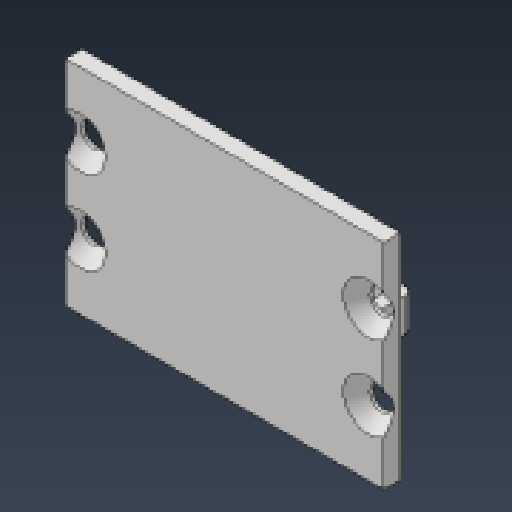
# Autodesk Inventor part: PCBs_Holder
Saved by Autodesk Inventor 2026.2 (Build 302298010, 298A)
## iProperties
Created: 2026-04-14
Part Number: PCBs_Holder
Material: Generic
Document SubType Name: Modeling
Designer: szymo
Density: 1 g/cm^3
Appearance: Default
Author: szymo
Autodesk Inventor part; units mm, degrees
ref_plane "YZ Plane" through (0, 0, 0) normal (1, 0, 0) x (0, 1, 0)
ref_plane "XZ Plane" through (0, 0, 0) normal (0, 1, 0) x (-1, 0, 0)
ref_plane "XY Plane" through (0, 0, 0) normal (0, 0, 1) x (1, 0, 0)
sketch "Sketch1" plane through (0, 0, 0) normal (0, 0, 1) x (1, 0, 0)
  line L0 (19.2, 22.3883) -> (-19.2, 22.3883)
  line L1 (-19, 22.3883) -> (-19, 47.9488)
  line L2 (-19.2, 47.9488) -> (19.2, 47.9488)
  line L3 (19, 47.9488) -> (19, 22.3883)
  line L4 (15, 33.1685) -> (9.5, 33.1685)
  line L5 (9.5, 33.1685) -> (9.5, 37.1685)
  line L6 (9.5, 37.1685) -> (15, 37.1685)
  line L7 (15, 37.1685) -> (15, 33.1685)
  line L8 (-15, 33.1685) -> (-9.5, 33.1685)
  line L9 (-9.5, 33.1685) -> (-9.5, 37.1685)
  line L10 (-9.5, 37.1685) -> (-15, 37.1685)
  line L11 (-15, 37.1685) -> (-15, 33.1685)
  circle A0 centre (-17.2, 40.1685) radius 1.75 projected
  circle A1 centre (-17.2, 30.1685) radius 1.75 projected
  line L12 (-19.2, 22.3883) -> (-15.2, 22.3883) projected
  line L13 (-15.2, 22.3883) -> (-15.2, 47.9488) projected
  line L14 (-19.2, 47.9488) -> (-15.2, 47.9488) projected
  line L15 (-19.2, 22.3883) -> (-19.2, 47.9488) projected
  circle A2 centre (17.2, 40.1685) radius 1.75 projected
  circle A3 centre (17.2, 30.1685) radius 1.75 projected
  line L16 (19.2, 22.3883) -> (15.2, 22.3883) projected
  line L17 (19.2, 22.3883) -> (19.2, 47.9488) projected
  line L18 (19.2, 47.9488) -> (15.2, 47.9488) projected
  line L19 (15.2, 22.3883) -> (15.2, 47.9488) projected
  point P0 (0, 0)
  dimension "d4" = 10.7802
  dimension "d5" = 10.7802
  dimension "d6" = 10.7802
  dimension "d7" = 10.7802
  dimension "d10" = 4
  dimension "d11" = 4
  dimension "d12" = 5.5
  dimension "d13" = 5.5
  dimension "d33" = 0.2
  dimension "d34" = 0.2
  dimension "d43" = 0.2
  dimension "d44" = 0.2
  constraints: 24 end point, 6 parallel, 4 coincident, 3 horizontal, 3 perpendicular, 3 point on line
  measures "d4" distance between parallel lines of L0 L4
  measures "d5" distance between parallel lines of L0 L8
  measures "d6" distance between parallel lines of L2 L6
  measures "d7" distance between parallel lines of L2 L10
  measures "d10" distance between parallel lines of L6 L4
  measures "d11" distance between parallel lines of L10 L8
  measures "d12" distance between parallel lines of L7 L5
  measures "d13" distance between parallel lines of L9 L11
  measures "d33" distance between parallel lines of L13 L11
  measures "d34" distance between parallel lines of L19 L7
  measures "d43" distance between parallel lines of L1 L15
  measures "d44" distance between parallel lines of L17 L3
extrude "Extrusion3" add sketch "Sketch1" against normal blind 2 contours L0 L19 L2 L3 | L0 L13 L2 L19 | L0 L1 L2 L13 | L4 L5 L6 L7 | L11 L10 L9 L8 | A0 | A1 | A2 | A3
extrude "Extrusion4" add sketch "Sketch1" against normal blind 7.5 contours L4 L5 L6 L7 | L11 L10 L9 L8
hole "Hole2" at (-17.2, 40.1685, 0) at (-17.2, 30.1685, 0) at (17.2, 40.1685, 0) at (17.2, 30.1685, 0) direction (0, 0, -1) diameter 2.9 end through all countersink diameter 6 countersink angle 90 clearance for "Countersunk Flat Head Screw ISO 2009/7046" size "M2.5" standard "ISO"
sketch "Sketch3" plane through (9.5, 33.1685, -2) normal (0, -1, 0) x (1, 0, 0)
  line L0 (0, 0) -> (0, -5.5) projected
  line L1 (5.5, -5.5) -> (0, -5.5) projected
  line L2 (5.5, 0) -> (5.5, -5.5) projected
  line L3 (-24.5, 0) -> (-24.5, -5.5) projected
  line L4 (-19, -5.5) -> (-24.5, -5.5) projected
  line L5 (-19, 0) -> (-19, -5.5) projected
  line L6 (5.5, 0) -> (5.5, -5.5) projected
  line L7 (5.5, -5.5) -> (0, 0)
  line L8 (5.5, 0) -> (0, -5.5)
  line L9 (-19, -5.5) -> (-24.5, 0)
  line L10 (-24.5, -5.5) -> (-19, 0)
  line L11 (-24.5, 0) -> (-19, 0) projected
  line L12 (0, 0) -> (5.5, 0) projected
  point P0 (-9.5, 2)
  point P1 (2.75, -2.75)
  point P2 (-21.75, -2.75)
  constraints: 8 end point, 3 perpendicular, 2 midpoint
hole "Hole3" at (12.25, 33.1685, -4.75) at (-12.25, 33.1685, -4.75) direction (0, 1, 0) diameter 2.5 end through all
fillet "Fillet2" radius 1 4 edges at (15, 35.1685, -7.5) (9.5, 35.1685, -7.5) (-9.5, 35.1685, -7.5) (-15, 35.1685, -7.5)
equation "\"d4\" = d6"
equation "\"d5\" = d7"
equation "\"d11\" = d10"
equation "\"d13\" = d12"
body "Solid2"
